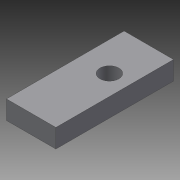
# Autodesk Inventor part: Effector_ZProbe_B
Saved by Autodesk Inventor 2014 (Build 180170000, 170)
## iProperties
Created: 2014-08-28
Part Number: Effector_ZProbe_B
Material: Generic
Document SubType Name: Modeling
Designer: ThatOtherGuy
Density: 1 g/cm^3
Appearance: Default
Author: ThatOtherGuy
Autodesk Inventor part; units mm, degrees
ref_plane "YZ Plane" through (0, 0, 0) normal (1, 0, 0) x (0, 1, 0)
ref_plane "XZ Plane" through (0, 0, 0) normal (0, 1, 0) x (-1, 0, 0)
ref_plane "XY Plane" through (0, 0, 0) normal (0, 0, 1) x (1, 0, 0)
sketch "Sketch1" plane through (0, 0, 0) normal (0, 0, 1) x (1, 0, 0)
  line L0 (0, 20) -> (0, 0)
  circle A0 centre (5, 12.5) radius 1.6
  line L1 (8.4, 20) -> (8.4, 0)
  line L2 (0, 20) -> (8.4, 20)
  line L3 (0, 0) -> (8.4, 0)
  dimension "d2" = 3.2
  dimension "d3" = 5
  dimension "d12" = 8.4
  dimension "d14" = 7.5
  dimension "d15" = 8.4
  dimension "d16" = 20
  constraints: 8 end point, 1 centre point, 1 coincident, 1 horizontal, 1 perpendicular
  measures "d2" diameter of A0
  measures "d3" distance from line of L0 A0.centre
  measures "d12" distance between parallel lines of L0 L1
  measures "d14" distance from line of L2 A0.centre
  measures "d15" distance of L0.start L1.start
  measures "d16" distance of L0.start L0.end
extrude "Extrusion1" add sketch "Sketch1" along normal blind 3.175
equation "\"d12\" = d13"
equation "\"d13\" = 8.4"
body "Solid1"
